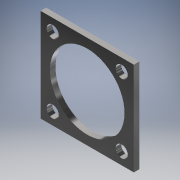
# Autodesk Inventor part: Pneumatic Upper Support
Saved by Autodesk Inventor 2019.4 (Build 234330000, 330)
## iProperties
Created: 2020-01-11
Part Number: Pneumatic Upper Support
Material: Aluminum 6061
Document SubType Name: Modeling
Designer: Mark
Mass: 15.2756 g
Surface Area: 50.2419 cm^2
Volume: 5.65762 cm^3
Density: 2.7 g/cm^3
Appearance: Aluminum - Flat
Author: Mark
Autodesk Inventor part; units mm, degrees
ref_plane "YZ Plane" through (0, 0, 0) normal (1, 0, 0) x (0, 1, 0)
ref_plane "XZ Plane" through (0, 0, 0) normal (0, 1, 0) x (-1, 0, 0)
ref_plane "XY Plane" through (0, 0, 0) normal (0, 0, 1) x (1, 0, 0)
sketch "Sketch1" plane through (0, 0, 0) normal (0, 0, 1) x (1, 0, 0)
  line L0 (-25, -25) -> (25, -25)
  line L1 (25, -25) -> (25, 25)
  line L2 (25, 25) -> (-25, 25)
  line L3 (-25, 25) -> (-25, -25)
  line L4 (-25, -25) -> (25, 25) construction
  line L5 (25, -25) -> (-25, 25) construction
  line L6 (-18.5, -18.5) -> (18.5, -18.5) construction
  line L7 (18.5, -18.5) -> (18.5, 18.5) construction
  line L8 (18.5, 18.5) -> (-18.5, 18.5) construction
  line L9 (-18.5, 18.5) -> (-18.5, -18.5) construction
  line L10 (-18.5, -18.5) -> (18.5, 18.5) construction
  line L11 (18.5, -18.5) -> (-18.5, 18.5) construction
  circle A0 centre (-18.5, 18.5) radius 3.25
  circle A1 centre (18.5, 18.5) radius 3.25
  circle A2 centre (18.5, -18.5) radius 3.25
  circle A3 centre (-18.5, -18.5) radius 3.25
  circle A4 centre (0, 0) radius 19
  dimension "d0" = 50
  dimension "d1" = 50
  dimension "d2" = 37
  dimension "d3" = 37
  dimension "d4" = 6.5
  dimension "d5" = 6.5
  dimension "d6" = 6.5
  dimension "d7" = 6.5
  dimension "d10" = 38
  constraints: 24 end point, 5 centre point, 5 coincident, 4 midpoint, 4 parallel, 2 horizontal, 2 perpendicular
  measures "d0" distance of L2.end L1.end
  measures "d1" distance of L1.end L0.end
  measures "d2" distance of L8.end L7.end
  measures "d3" distance of L7.end L6.end
  measures "d4" diameter of A0
  measures "d5" diameter of A1
  measures "d6" diameter of A2
  measures "d7" diameter of A3
  measures "d10" diameter of A4
extrude "Extrusion1" add sketch "Sketch1" along normal blind 3
sketch "Sketch2" plane through (0, 0, 0) normal (0, 0, -1) x (-1, 0, 0)
  line L0 (-25, 25) -> (25, 25) projected
  line L1 (10, 25) -> (-10, 25)
  line L2 (-10, 25) -> (-10, 22)
  line L3 (-10, 22) -> (10, 22)
  line L4 (10, 22) -> (10, 25)
  line L5 (-25, -25) -> (-25, 25) projected
  point P0 (0, 0)
  dimension "d11" = 20
  dimension "d12" = 3
  dimension "d13" = 15
  constraints: 8 end point, 2 parallel, 1 horizontal, 1 perpendicular, 1 point on line
  measures "d11" distance of L3.end L2.end
  measures "d12" distance of L2.end L1.end
  measures "d13" distance between parallel lines of L5 L2
extrude "Extrusion2" add sketch "Sketch2" along normal blind 30
fillet "Fillet1" radius 8 1 edges at (0, 22, 0)
sketch "Sketch3" plane through (-10, 22, -30) normal (0, -1, 0) x (1, 0, 0)
  circle A0 centre (10, 5) radius 2.75
  circle A1 centre (15, 15) radius 2.75
  line L0 (20, 0) -> (0, 0) projected
  line L1 (0, 22.2041) -> (0, 0) projected
  line L2 (20, 22.2041) -> (20, 0) projected
  line L3 (-15, 30) -> (35, 30) projected
  point P0 (10, 30)
  dimension "d17" = 5.5
  dimension "d18" = 5.5
  dimension "d19" = 5
  dimension "d20" = 10
  dimension "d21" = 5
  dimension "d22" = 15
  constraints: 2 centre point
  measures "d17" diameter of A0
  measures "d18" diameter of A1
  measures "d19" distance from line of L0 A0.centre
  measures "d20" distance from line of L1 A0.centre
  measures "d21" distance from line of L2 A1.centre
  measures "d22" distance from line of L3 A1.centre
extrude "Extrusion3" cut sketch "Sketch3" against normal blind 30
body "Solid1"
